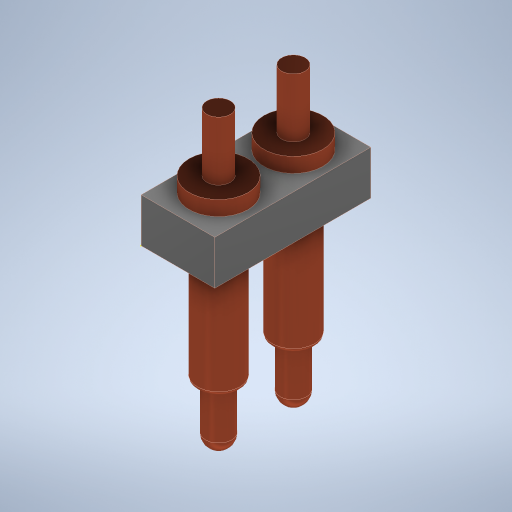
# Autodesk Inventor part: Pogo_Pin
Saved by Autodesk Inventor 2024 (Build 280153000, 153)
## iProperties
Created: 2023-11-13
Part Number: Pogo_Pin
Material: 铜
Document SubType Name: Modeling
Designer: lunima
Density: 8.94 g/cm^3
Appearance: 铜 - 缎光
Author: lunima
Autodesk Inventor part; units mm, degrees
ref_plane "YZ Plane" through (0, 0, 0) normal (1, 0, 0) x (0, 1, 0)
ref_plane "XZ Plane" through (0, 0, 0) normal (0, 1, 0) x (-1, 0, 0)
ref_plane "XY Plane" through (0, 0, 0) normal (0, 0, 1) x (1, 0, 0)
sketch "草图1" plane through (0, 0, 0) normal (0, 1, 0) x (-1, 0, 0)
  point P0 (0, 0)
sketch "草图2" plane through (0, 0, 0) normal (0, 1, 0) x (-1, 0, 0)
  line L0 (0, 0) -> (-2.5, 0)
  line L1 (-2.5, 0) -> (-2.5, -5.3)
  line L2 (-2.5, -5.3) -> (0, -5.3)
  line L3 (0, -5.3) -> (0, 0)
  dimension "d0" = 2.5
  dimension "d1" = 5.3
  constraints: 8 end point, 2 parallel, 1 horizontal, 1 perpendicular
  measures "d0" distance of L2.end L1.end
  measures "d1" distance of L1.end L0.end
extrude "拉伸1" add sketch "草图2" along normal blind 1.5
sketch "草图3" plane through (0, 1.5, 0) normal (0, 1, 0) x (1, 0, 0)
  line L0 (2.5, 5.3) -> (0, 5.3) projected
  line L1 (1.25, 5.3) -> (1.25, 0)
  line L2 (0, 5.3) -> (0, 0) projected
  line L3 (1.25, 2.65) -> (1.25, 3.92)
  line L4 (1.25, 3.92) -> (1.25, 1.38)
  circle A0 centre (1.25, 3.92) radius 1
  circle A1 centre (1.25, 1.38) radius 1
  dimension "d4" = 1.27
  dimension "d5" = 2.54
  dimension "d6" = 2
  dimension "d7" = 2
  constraints: 6 end point, 2 centre point, 2 coincident, 2 midpoint, 2 point on line, 1 parallel
  measures "d4" distance of L3.start L3.end
  measures "d5" distance of L3.end L4.end
  measures "d6" diameter of A0
  measures "d7" diameter of A1
extrude "拉伸2" add sketch "草图3" along normal blind 0.5
sketch "草图4" plane through (1.25, 2, -1.38) normal (0, 1, 0) x (1, 0, 0)
  circle A0 centre (0, 0) radius 0.4
  circle A1 centre (0, 2.54) radius 1 projected
  circle A2 centre (0, 2.54) radius 0.4
  point P0 (-1.25, -1.38)
  dimension "d10" = 0.8
  dimension "d11" = 0.8
  constraints: 2 centre point, 1 coincident
  measures "d10" diameter of A0
  measures "d11" diameter of A2
extrude "拉伸3" add sketch "草图4" along normal blind 2 contours A0 | A2
sketch "草图5" plane through (0, 0, 0) normal (0, -1, 0) x (1, 0, 0)
  circle A0 centre (1.25, -3.92) radius 0.4 projected
  circle A1 centre (1.25, -3.92) radius 0.725
  circle A2 centre (1.25, -1.38) radius 0.4 projected
  circle A3 centre (1.25, -1.38) radius 0.725
  point P0 (0, 0)
  dimension "d14" = 1.45
  dimension "d15" = 1.45
  constraints: 2 centre point, 2 coincident
  measures "d14" diameter of A1
  measures "d15" diameter of A3
extrude "拉伸4" add sketch "草图5" along normal blind 4 contours A0 | A1 | A2 | A3
sketch "草图6" plane through (1.25, -4, -1.38) normal (0, -1, 0) x (1, 0, 0)
  circle A0 centre (0, 0) radius 0.45
  circle A1 centre (0, -2.54) radius 0.725 projected
  circle A2 centre (0, -2.54) radius 0.45
  point P0 (-1.25, 1.38)
  dimension "d18" = 0.9
  dimension "d19" = 0.9
  constraints: 2 centre point, 1 coincident
  measures "d18" diameter of A0
  measures "d19" diameter of A2
extrude "拉伸5" add sketch "草图6" along normal blind 2 contours A0 | A2
fillet "圆角1" radius 0.45 1 edges at (0.8, -6, -3.92)
fillet "圆角2" radius 0.45 1 edges at (0.8, -6, -1.38)
fillet "圆角3" radius 0.15 2 edges at (0.525, -4, -3.92) (0.525, -4, -1.38)
